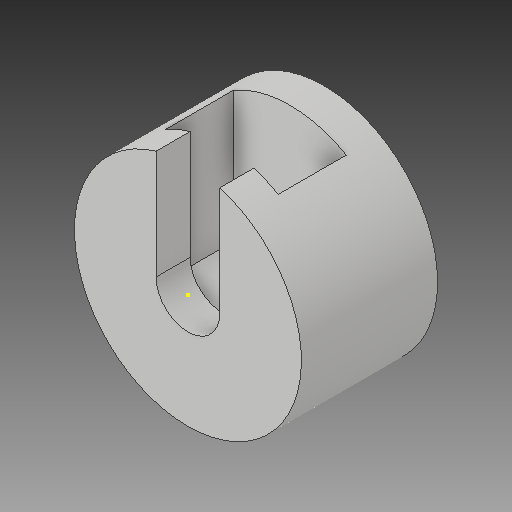
# Autodesk Inventor part: Acople tornillo M8
Saved by Autodesk Inventor 2019 (Build 230136000, 136)
## iProperties
Created: 2020-02-01
Part Number: Acople tornillo M8
Material: Generic
Document SubType Name: Modeling
Designer: Elías Sánchez
Density: 1 g/cm^3
Appearance: Default
Description: Impresión 3D
Author: Elías Sánchez
Revision Number: IR
Autodesk Inventor part; units mm, degrees
ref_plane "YZ Plane" through (0, 0, 0) normal (1, 0, 0) x (0, 1, 0)
ref_plane "XZ Plane" through (0, 0, 0) normal (0, 1, 0) x (-1, 0, 0)
sketch "Sketch1" plane through (0, 0, 0) normal (0, 0, 1) x (1, 0, 0)
  point P0 (0, 0)
sketch "Sketch2" plane through (0, 0, 0) normal (0, 0, 1) x (1, 0, 0)
  circle A0 centre (0, 0) radius 12.5
  dimension "d0" = 25
  constraints: 1 centre point, 1 coincident
  measures "d0" diameter of A0
extrude "Extrusion1" add sketch "Sketch2" along normal blind 15
ref_plane "Work Plane1" through (0, 0, 7.5) normal (0, 0, 1) x (1, 0, 0)
sketch "Sketch3" plane through (0, 0, 7.5) normal (0, 0, 1) x (1, 0, 0)
  line L0 (6.2, -3.5796) -> (0, -7.1591)
  line L1 (0, -7.1591) -> (-6.2, -3.5796)
  line L2 (-6.2, -3.5796) -> (-6.2, 3.5796)
  line L3 (-6.2, 3.5796) -> (0, 7.1591)
  line L4 (0, 7.1591) -> (6.2, 3.5796)
  line L5 (6.2, 3.5796) -> (6.2, -3.5796)
  point P0 (0, 0)
  point P1 (0, 0)
  dimension "d4" = 12.4
  constraints: 12 end point, 2 coincident, 1 vertical, 13 other
  measures "d4" distance between parallel lines of L5 L2
extrude "Extrusion2" cut sketch "Sketch3" along normal mid plane 7.5
sketch "Sketch4" plane through (0, 0, 0) normal (0, 1, 0) x (-1, 0, 0)
  line L0 (6.2, 11.25) -> (0, 11.25) projected
  line L1 (-6.2, 3.75) -> (0, 3.75) projected
  line L2 (6.2, 11.25) -> (-6.2, 11.25)
  line L3 (-6.2, 11.25) -> (-6.2, 3.75)
  line L4 (-6.2, 3.75) -> (6.2, 3.75)
  line L5 (6.2, 3.75) -> (6.2, 11.25)
  point P0 (0, 0)
  constraints: 8 end point, 2 parallel, 1 horizontal, 1 perpendicular
extrude "Extrusion3" cut sketch "Sketch4" along normal blind 15
sketch "Sketch5" plane through (0, 0, 15) normal (0, 0, 1) x (1, 0, 0)
  circle A0 centre (0, 0) radius 12.5 projected
  constraints: 1 coincident
hole "Hole1" at (0, 0, 15) direction (0, 0, -1) diameter 7 depth 7.5
sketch "Sketch6" plane through (0, 0, 15) normal (0, 0, 1) x (1, 0, 0)
  point P0 (0, 0)
sketch "Sketch7" plane through (0, 0, 0) normal (0, 1, 0) x (-1, 0, 0)
  line L0 (3.5, 11.25) -> (-3.5, 11.25) projected
  line L1 (-3.5, 15) -> (3.5, 15) projected
  line L2 (3.5, 11.25) -> (-3.5, 11.25)
  line L3 (-3.5, 11.25) -> (-3.5, 15)
  line L4 (-3.5, 15) -> (3.5, 15)
  line L5 (3.5, 15) -> (3.5, 11.25)
  point P0 (0, 0)
  constraints: 8 end point, 2 parallel, 1 horizontal, 1 perpendicular
extrude "Extrusion4" cut sketch "Sketch7" along normal blind 15
body "Solid1"
